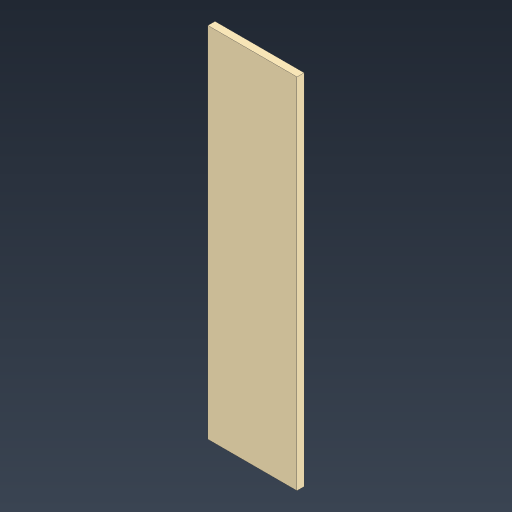
# Autodesk Inventor part: Вертикальная_поверхность
Saved by Autodesk Inventor 2023.2 (Build 272271030, 271C)
## iProperties
Created: 2025-12-05
Part Number: Вертикальная_поверхность
Material: Типовые
Document SubType Name: Modeling
Designer: Олег Коноваленко
Density: 1 g/cm^3
Appearance: По умолчанию
Author: Олег Коноваленко
Autodesk Inventor part; units mm, degrees
ref_plane "YZ Plane" through (0, 0, 0) normal (1, 0, 0) x (0, 1, 0)
ref_plane "XZ Plane" through (0, 0, 0) normal (0, 1, 0) x (-1, 0, 0)
ref_plane "XY Plane" through (0, 0, 0) normal (0, 0, 1) x (1, 0, 0)
sketch "Эскиз1" plane through (0, 0, 0) normal (0, 0, 1) x (1, 0, 0)
  line L0 (-100, -402.124) -> (100, -402.124)
  line L1 (100, -402.124) -> (100, 402.124)
  line L2 (100, 402.124) -> (-100, 402.124)
  line L3 (-100, 402.124) -> (-100, -402.124)
  line L4 (-100, -402.124) -> (100, 402.124) construction
  line L5 (100, -402.124) -> (-100, 402.124) construction
  point P0 (0, 0)
  dimension "d0" = 804.248
  dimension "d1" = 200
  constraints: 12 end point, 2 midpoint, 2 parallel, 1 horizontal, 1 perpendicular
  measures "d0" distance of L0.end L1.end
  measures "d1" distance of L0.start L0.end
extrude "Выдавливание1" add sketch "Эскиз1" along normal mid plane 16
